Autodesk Fusion 360 part; units mm, degrees
(part 9 of 9)
fillet "Fillet15" radius 1 34 edges at (252.5312, 2.1, 39.625) (247.5312, 2.1, 39.625) (252.5312, 2.1, 55.625) (247.5312, 2.1, 55.625) (226.3375, 2.1, 55.625) (221.3375, 2.1, 55.625) (226.3375, 2.1, 39.625) (221.3375, 2.1, 39.625) (207.2875, 2.1, 55.625) (202.2875, 2.1, 55.625) (207.2875, 2.1, 39.625) (202.2875, 2.1, 39.625) (188.2375, 2.1, 55.625) (183.2375, 2.1, 55.625) (188.2375, 2.1, 39.625) (183.2375, 2.1, 39.625) (169.1875, 2.1, 39.625) (164.1875, 2.1, 39.625) (150.1375, 2.1, 39.625) (145.1375, 2.1, 39.625) (131.0875, 2.1, 39.625) (126.0875, 2.1, 39.625) (112.0375, 2.1, 39.625) (107.0375, 2.1, 39.625) (92.9875, 2.1, 39.625) (87.9875, 2.1, 39.625) (73.9375, 2.1, 39.625) (68.9375, 2.1, 39.625) (73.9375, 2.1, 55.625) (68.9375, 2.1, 55.625) (54.8875, 2.1, 55.625) (49.8875, 2.1, 55.625) (54.8875, 2.1, 39.625) (49.8875, 2.1, 39.625)
fillet "Fillet16" radius 1 64 edges at (45.3625, 2.1, 20.575) (40.3625, 2.1, 20.575) (35.6, 2.1, 17.525) (40.6, 2.1, 17.525) (35.6, 2.1, 1.525) (40.6, 2.1, 1.525) (54.65, 2.1, 17.525) (59.65, 2.1, 17.525) (59.4125, 2.1, 20.575) (64.4125, 2.1, 20.575) (54.65, 2.1, 1.525) (59.65, 2.1, 1.525) (78.4625, 2.1, 20.575) (83.4625, 2.1, 20.575) (73.7, 2.1, 17.525) (78.7, 2.1, 17.525) (73.7, 2.1, 1.525) (78.7, 2.1, 1.525) (97.5125, 2.1, 20.575) (102.5125, 2.1, 20.575) (92.75, 2.1, 17.525) (97.75, 2.1, 17.525) (92.75, 2.1, 1.525) (97.75, 2.1, 1.525) (116.5625, 2.1, 20.575) (121.5625, 2.1, 20.575) (111.8, 2.1, 17.525) (116.8, 2.1, 17.525) (111.8, 2.1, 1.525) (116.8, 2.1, 1.525) (135.6125, 2.1, 20.575) (140.6125, 2.1, 20.575) (130.85, 2.1, 17.525) (135.85, 2.1, 17.525) (130.85, 2.1, 1.525) (135.85, 2.1, 1.525) (154.6625, 2.1, 20.575) (159.6625, 2.1, 20.575) (149.9, 2.1, 17.525) (154.9, 2.1, 17.525) (149.9, 2.1, 1.525) (154.9, 2.1, 1.525) (173.7125, 2.1, 20.575) (178.7125, 2.1, 20.575) (168.95, 2.1, 17.525) (173.95, 2.1, 17.525) (168.95, 2.1, 1.525) (173.95, 2.1, 1.525) (192.7625, 2.1, 20.575) (197.7625, 2.1, 20.575) (188, 2.1, 17.525) (193, 2.1, 17.525) (188, 2.1, 1.525) (193, 2.1, 1.525) (211.8125, 2.1, 20.575) (216.8125, 2.1, 20.575) (207.05, 2.1, 17.525) (212.05, 2.1, 17.525) (207.05, 2.1, 1.525) (212.05, 2.1, 1.525) (230.8625, 2.1, 1.525) (235.8625, 2.1, 1.525) (254.675, 2.1, 1.525) (259.675, 2.1, 1.525)
fillet "Fillet17" radius 1 18 edges at (59.4125, 2.1, 36.575) (64.4125, 2.1, 36.575) (78.4625, 2.1, 36.575) (83.4625, 2.1, 36.575) (97.5125, 2.1, 36.575) (102.5125, 2.1, 36.575) (116.5625, 2.1, 36.575) (121.5625, 2.1, 36.575) (135.6125, 2.1, 36.575) (140.6125, 2.1, 36.575) (154.6625, 2.1, 36.575) (159.6625, 2.1, 36.575) (173.7125, 2.1, 36.575) (178.7125, 2.1, 36.575) (192.7625, 2.1, 36.575) (197.7625, 2.1, 36.575) (211.8125, 2.1, 36.575) (216.8125, 2.1, 36.575)
sketch "Sketch15" plane through (0, 0, 0) normal (0, -1, 0) x (1, 0, 0)
  line L0 (6.3312, 56.625) -> (10.5375, 56.625)
  arc A0 (10.5375, 56.625) -> (11.05, 58.15) centre (8.525, 58.15) ccw
  line L1 (11.05, 58.15) -> (11.05, 73.2)
  arc A1 (12.525, 74.675) -> (11.05, 73.2) centre (12.525, 73.2) ccw
  line L2 (12.525, 74.675) -> (91.0563, 74.675)
  arc A2 (92.0563, 75.675) -> (91.0563, 74.675) centre (92.0563, 74.675) ccw
  line L3 (92.0563, 75.675) -> (98.0563, 75.675)
  arc A3 (99.0563, 74.675) -> (98.0563, 75.675) centre (98.0563, 74.675) ccw
  line L4 (99.0563, 74.675) -> (115.2563, 74.675)
  arc A4 (116.2563, 75.675) -> (115.2563, 74.675) centre (116.2563, 74.675) ccw
  line L5 (116.2563, 75.675) -> (122.2563, 75.675)
  arc A5 (123.2563, 74.675) -> (122.2563, 75.675) centre (122.2563, 74.675) ccw
  line L6 (123.2563, 74.675) -> (131.5375, 74.675)
  arc A6 (132.5375, 75.675) -> (131.5375, 74.675) centre (132.5375, 74.675) ccw
  line L7 (132.5375, 75.675) -> (138.5375, 75.675)
  arc A7 (139.5375, 74.675) -> (138.5375, 75.675) centre (138.5375, 74.675) ccw
  line L8 (139.5375, 74.675) -> (155.7375, 74.675)
  arc A8 (156.7375, 75.675) -> (155.7375, 74.675) centre (156.7375, 74.675) ccw
  line L9 (156.7375, 75.675) -> (162.7375, 75.675)
  arc A9 (163.7375, 74.675) -> (162.7375, 75.675) centre (162.7375, 74.675) ccw
  line L10 (163.7375, 74.675) -> (239.8875, 74.675)
  arc A10 (241.3625, 73.2) -> (239.8875, 74.675) centre (239.8875, 73.2) ccw
  line L11 (241.3625, 73.2) -> (241.3625, 58.15)
  arc A11 (241.3625, 58.15) -> (243.8875, 55.625) centre (243.8875, 58.15) ccw
  line L12 (243.8875, 55.625) -> (263.7, 55.625)
  arc A12 (265.175, 54.15) -> (263.7, 55.625) centre (263.7, 54.15) ccw
  line L13 (265.175, 54.15) -> (265.175, 3)
  arc A13 (263.7, 1.525) -> (265.175, 3) centre (263.7, 3) ccw
  line L14 (263.7, 1.525) -> (3, 1.525)
  arc A14 (1.525, 3) -> (3, 1.525) centre (3, 3) ccw
  line L15 (1.525, 3) -> (1.525, 54.15)
  arc A15 (3, 55.625) -> (1.525, 54.15) centre (3, 54.15) ccw
  line L16 (3, 55.625) -> (5.3312, 55.625)
  arc A16 (6.3312, 56.625) -> (5.3312, 55.625) centre (6.3312, 55.625) ccw
  arc A17 (266.7, 54.15) -> (263.7, 57.15) centre (263.7, 54.15) ccw
  line L17 (263.7, 57.15) -> (243.8875, 57.15)
  arc A18 (242.8875, 58.15) -> (243.8875, 57.15) centre (243.8875, 58.15) ccw
  line L18 (242.8875, 58.15) -> (242.8875, 73.2)
  arc A19 (242.8875, 73.2) -> (239.8875, 76.2) centre (239.8875, 73.2) ccw
  line L19 (239.8875, 76.2) -> (12.525, 76.2)
  arc A20 (12.525, 76.2) -> (9.525, 73.2) centre (12.525, 73.2) ccw
  line L20 (9.525, 73.2) -> (9.525, 58.15)
  arc A21 (8.525, 57.15) -> (9.525, 58.15) centre (8.525, 58.15) ccw
  line L21 (8.525, 57.15) -> (3, 57.15)
  arc A22 (3, 57.15) -> (0, 54.15) centre (3, 54.15) ccw
  line L22 (0, 54.15) -> (0, 3)
  arc A23 (0, 3) -> (3, 0) centre (3, 3) ccw
  line L23 (3, 0) -> (263.7, 0)
  arc A24 (263.7, 0) -> (266.7, 3) centre (263.7, 3) ccw
  line L24 (266.7, 3) -> (266.7, 54.15)
  line L25 (91.0563, 73.675) -> (99.0563, 73.675)
  line L26 (99.0563, 73.675) -> (99.0563, 76.2)
  line L27 (99.0563, 76.2) -> (91.0563, 76.2)
  line L28 (91.0563, 76.2) -> (91.0563, 73.675)
  line L29 (91.0563, 72.675) -> (91.0563, 74.675)
  line L30 (115.2563, 73.9823) -> (123.2563, 73.9823)
  line L31 (123.2563, 73.9823) -> (123.2563, 77)
  line L32 (123.2563, 77) -> (115.2563, 77)
  line L33 (115.2563, 77) -> (115.2563, 73.9823)
  line L34 (115.2563, 73.675) -> (115.2563, 74.675)
  line L35 (131.5375, 74.2141) -> (139.5375, 74.2141)
  line L36 (139.5375, 74.2141) -> (139.5375, 77.289)
  line L37 (139.5375, 77.289) -> (131.5375, 77.289)
  line L38 (131.5375, 77.289) -> (131.5375, 74.2141)
  line L39 (131.5375, 74.675) -> (131.5375, 62.425)
  line L40 (155.7375, 74.3532) -> (163.7375, 74.3532)
  line L41 (163.7375, 74.3532) -> (163.7375, 77.2272)
  line L42 (163.7375, 77.2272) -> (155.7375, 77.2272)
  line L43 (155.7375, 77.2272) -> (155.7375, 74.3532)
  line L44 (155.7375, 73.675) -> (155.7375, 74.675)
  dimension "d416" = 8
  dimension "d417" = 8
  dimension "d418" = 8
  dimension "d419" = 8
  constraint horizontal L25
  constraint vertical L26
  constraint horizontal L27
  constraint vertical L28
  constraint coincident L19 L26.end
  constraint midpoint L25.start L29
  constraint horizontal L30
  constraint vertical L31
  constraint horizontal L32
  constraint vertical L33
  constraint coincident L30.start L34
  constraint horizontal L35
  constraint vertical L36
  constraint horizontal L37
  constraint vertical L38
  constraint coincident L35.start L39
  constraint horizontal L40
  constraint vertical L41
  constraint horizontal L42
  constraint vertical L43
  constraint coincident L40.start L44
  measures "d416" distance of L26.end L27.end
  measures "d417" distance of L31.end L32.end
  measures "d418" distance of L36.end L37.end
  measures "d419" distance of L41.end L42.end
extrude "Extrude14" cut sketch "Sketch15" against normal blind 3.6 contours A2 L3 A3 L19 L26 L27 L28 | A4 L5 A5 L19 L31 L33 | A6 L7 A7 L19 L36 L38 | A8 L9 A9 L19 L41 L43
sketch "Sketch16" plane through (0, 0, 0) normal (0, -1, 0) x (1, 0, 0)
  line L0 (163.7375, 76.2) -> (163.7375, 74.675)
  line L1 (163.7375, 74.675) -> (239.8875, 74.675)
  arc A0 (241.3625, 73.2) -> (239.8875, 74.675) centre (239.8875, 73.2) ccw
  line L2 (241.3625, 73.2) -> (241.3625, 58.15)
  arc A1 (241.3625, 58.15) -> (243.8875, 55.625) centre (243.8875, 58.15) ccw
  line L3 (243.8875, 55.625) -> (263.7, 55.625)
  arc A2 (265.175, 54.15) -> (263.7, 55.625) centre (263.7, 54.15) ccw
  line L4 (265.175, 54.15) -> (265.175, 3)
  arc A3 (263.7, 1.525) -> (265.175, 3) centre (263.7, 3) ccw
  line L5 (263.7, 1.525) -> (3, 1.525)
  arc A4 (1.525, 3) -> (3, 1.525) centre (3, 3) ccw
  line L6 (1.525, 3) -> (1.525, 54.15)
  arc A5 (3, 55.625) -> (1.525, 54.15) centre (3, 54.15) ccw
  line L7 (3, 55.625) -> (5.3312, 55.625)
  arc A6 (6.3312, 56.625) -> (5.3312, 55.625) centre (6.3312, 55.625) ccw
  line L8 (6.3312, 56.625) -> (10.5375, 56.625)
  arc A7 (10.5375, 56.625) -> (11.05, 58.15) centre (8.525, 58.15) ccw
  line L9 (11.05, 58.15) -> (11.05, 73.2)
  arc A8 (12.525, 74.675) -> (11.05, 73.2) centre (12.525, 73.2) ccw
  line L10 (12.525, 74.675) -> (91.0563, 74.675)
  line L11 (91.0563, 74.675) -> (91.0563, 76.2)
  line L12 (91.0563, 76.2) -> (12.525, 76.2)
  arc A9 (12.525, 76.2) -> (9.525, 73.2) centre (12.525, 73.2) ccw
  line L13 (9.525, 73.2) -> (9.525, 58.15)
  arc A10 (8.525, 57.15) -> (9.525, 58.15) centre (8.525, 58.15) ccw
  line L14 (8.525, 57.15) -> (3, 57.15)
  arc A11 (3, 57.15) -> (0, 54.15) centre (3, 54.15) ccw
  line L15 (0, 54.15) -> (0, 3)
  arc A12 (0, 3) -> (3, 0) centre (3, 3) ccw
  line L16 (3, 0) -> (263.7, 0)
  arc A13 (263.7, 0) -> (266.7, 3) centre (263.7, 3) ccw
  line L17 (266.7, 3) -> (266.7, 54.15)
  arc A14 (266.7, 54.15) -> (263.7, 57.15) centre (263.7, 54.15) ccw
  line L18 (263.7, 57.15) -> (243.8875, 57.15)
  arc A15 (242.8875, 58.15) -> (243.8875, 57.15) centre (243.8875, 58.15) ccw
  line L19 (242.8875, 58.15) -> (242.8875, 73.2)
  arc A16 (242.8875, 73.2) -> (239.8875, 76.2) centre (239.8875, 73.2) ccw
  line L20 (239.8875, 76.2) -> (163.7375, 76.2)
  line L21 (9.525, 60.8894) -> (5.3312, 60.8894)
  line L22 (5.3312, 60.8894) -> (5.3312, 53.9931)
  line L23 (5.3312, 53.9931) -> (9.525, 53.9931)
  line L24 (9.525, 53.9931) -> (9.525, 60.8894)
  line L25 (5.3312, 53.625) -> (5.3312, 55.625)
  constraint horizontal L21
  constraint vertical L22
  constraint horizontal L23
  constraint vertical L24
  constraint coincident L22.end L25
  constraint coincident L13 L21.start
extrude "Extrude15" cut sketch "Sketch16" against normal blind 3.6 contours A6 L8 A10 L14 L22 L24
